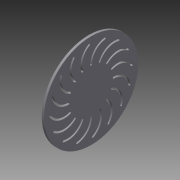
# Autodesk Inventor part: FanCentRotorRear
Saved by Autodesk Inventor 2018.2 (Build 222227000, 227)
## iProperties
Created: 2018-02-04
Part Number: FanCentRotorRear
Material: Generic
Document SubType Name: Sheet Metal
Designer: Rus
Density: 1 g/cm^3
Sheet Metal Rule: Default
Appearance: Default
Author: Rus
Autodesk Inventor part; units mm, degrees
ref_plane "YZ Plane" through (0, 0, 0) normal (1, 0, 0) x (0, 1, 0)
ref_plane "XZ Plane" through (0, 0, 0) normal (0, 1, 0) x (-1, 0, 0)
ref_plane "XY Plane" through (0, 0, 0) normal (0, 0, 1) x (1, 0, 0)
sketch "Sketch1" plane through (0, 0, 0) normal (1, 0, 0) x (0, 1, 0)
  circle A0 centre (0, 0) radius 63.5
  arc A1 (51.7144, -18.8225) -> (30.3724, 0) centre (30.3724, -21.5106) ccw construction
  arc A2 (52.8957, -18.6737) -> (30.3724, 1.1906) centre (30.3724, -21.5106) ccw
  arc A3 (50.5331, -18.9713) -> (30.3724, -1.1906) centre (30.3724, -21.5106) ccw
  arc A4 (50.5331, -18.9713) -> (52.8957, -18.6737) centre (51.7144, -18.8225) ccw
  arc A5 (30.3724, 1.1906) -> (30.3724, -1.1906) centre (30.3724, 0) ccw
  line L0 (51.7144, -18.8225) -> (59.6705, -21.7183) construction
  line L1 (30.3724, 0) -> (63.5, 0) construction
  arc A6 (54.981, 2.4005) -> (28.0605, 11.623) centre (36.2922, -8.2502) ccw construction
  arc A7 (56.0154, 2.99) -> (27.6048, 12.723) centre (36.2922, -8.2502) ccw
  arc A8 (53.9465, 1.811) -> (28.5161, 10.523) centre (36.2922, -8.2502) ccw
  arc A9 (53.9465, 1.811) -> (56.0154, 2.99) centre (54.981, 2.4005) ccw
  arc A10 (27.6048, 12.723) -> (28.5161, 10.523) centre (28.0605, 11.623) ccw
  line L2 (54.981, 2.4005) -> (63.4396, 2.7698) construction
  line L3 (28.0605, 11.623) -> (58.6664, 24.3004) construction
  arc A11 (49.8771, 23.2581) -> (21.4765, 21.4765) centre (36.6869, 6.2662) ccw construction
  arc A12 (50.6072, 24.1986) -> (20.6346, 22.3184) centre (36.6869, 6.2662) ccw
  arc A13 (49.147, 22.3176) -> (22.3184, 20.6346) centre (36.6869, 6.2662) ccw
  arc A14 (49.147, 22.3176) -> (50.6072, 24.1986) centre (49.8771, 23.2581) ccw
  arc A15 (20.6346, 22.3184) -> (22.3184, 20.6346) centre (21.4765, 21.4765) ccw
  line L4 (49.8771, 23.2581) -> (57.5505, 26.8363) construction
  line L5 (21.4765, 21.4765) -> (44.9013, 44.9013) construction
  arc A16 (37.18, 40.5748) -> (11.623, 28.0605) centre (31.4962, 19.8287) ccw construction
  arc A17 (37.4946, 41.7231) -> (10.523, 28.5161) centre (31.4962, 19.8287) ccw
  arc A18 (36.8654, 39.4265) -> (12.723, 27.6048) centre (31.4962, 19.8287) ccw
  arc A19 (36.8654, 39.4265) -> (37.4946, 41.7231) centre (37.18, 40.5748) ccw
  arc A20 (10.523, 28.5161) -> (12.723, 27.6048) centre (11.623, 28.0605) ccw
  line L6 (37.18, 40.5748) -> (42.9, 46.8171) construction
  line L7 (11.623, 28.0605) -> (24.3004, 58.6664) construction
  arc A21 (18.8225, 51.7144) -> (0, 30.3724) centre (21.5106, 30.3724) ccw construction
  arc A22 (18.6737, 52.8957) -> (-1.1906, 30.3724) centre (21.5106, 30.3724) ccw
  arc A23 (18.9713, 50.5331) -> (1.1906, 30.3724) centre (21.5106, 30.3724) ccw
  arc A24 (18.9713, 50.5331) -> (18.6737, 52.8957) centre (18.8225, 51.7144) ccw
  arc A25 (-1.1906, 30.3724) -> (1.1906, 30.3724) centre (0, 30.3724) ccw
  line L8 (18.8225, 51.7144) -> (21.7183, 59.6705) construction
  line L9 (0, 30.3724) -> (0, 63.5) construction
  arc A26 (-2.4005, 54.981) -> (-11.623, 28.0605) centre (8.2502, 36.2922) ccw construction
  arc A27 (-2.99, 56.0154) -> (-12.723, 27.6048) centre (8.2502, 36.2922) ccw
  arc A28 (-1.811, 53.9465) -> (-10.523, 28.5161) centre (8.2502, 36.2922) ccw
  arc A29 (-1.811, 53.9465) -> (-2.99, 56.0154) centre (-2.4005, 54.981) ccw
  arc A30 (-12.723, 27.6048) -> (-10.523, 28.5161) centre (-11.623, 28.0605) ccw
  line L10 (-2.4005, 54.981) -> (-2.7698, 63.4396) construction
  line L11 (-11.623, 28.0605) -> (-24.3004, 58.6664) construction
  arc A31 (-23.2581, 49.8771) -> (-21.4765, 21.4765) centre (-6.2662, 36.6869) ccw construction
  arc A32 (-24.1986, 50.6072) -> (-22.3184, 20.6346) centre (-6.2662, 36.6869) ccw
  arc A33 (-22.3176, 49.147) -> (-20.6346, 22.3184) centre (-6.2662, 36.6869) ccw
  arc A34 (-22.3176, 49.147) -> (-24.1986, 50.6072) centre (-23.2581, 49.8771) ccw
  arc A35 (-22.3184, 20.6346) -> (-20.6346, 22.3184) centre (-21.4765, 21.4765) ccw
  line L12 (-23.2581, 49.8771) -> (-26.8363, 57.5505) construction
  line L13 (-21.4765, 21.4765) -> (-44.9013, 44.9013) construction
  arc A36 (-40.5748, 37.18) -> (-28.0605, 11.623) centre (-19.8287, 31.4962) ccw construction
  arc A37 (-41.7231, 37.4946) -> (-28.5161, 10.523) centre (-19.8287, 31.4962) ccw
  arc A38 (-39.4265, 36.8654) -> (-27.6048, 12.723) centre (-19.8287, 31.4962) ccw
  arc A39 (-39.4265, 36.8654) -> (-41.7231, 37.4946) centre (-40.5748, 37.18) ccw
  arc A40 (-28.5161, 10.523) -> (-27.6048, 12.723) centre (-28.0605, 11.623) ccw
  line L14 (-40.5748, 37.18) -> (-46.8171, 42.9) construction
  line L15 (-28.0605, 11.623) -> (-58.6664, 24.3004) construction
  arc A41 (-51.7144, 18.8225) -> (-30.3724, 0) centre (-30.3724, 21.5106) ccw construction
  arc A42 (-52.8957, 18.6737) -> (-30.3724, -1.1906) centre (-30.3724, 21.5106) ccw
  arc A43 (-50.5331, 18.9713) -> (-30.3724, 1.1906) centre (-30.3724, 21.5106) ccw
  arc A44 (-50.5331, 18.9713) -> (-52.8957, 18.6737) centre (-51.7144, 18.8225) ccw
  arc A45 (-30.3724, -1.1906) -> (-30.3724, 1.1906) centre (-30.3724, 0) ccw
  line L16 (-51.7144, 18.8225) -> (-59.6705, 21.7183) construction
  line L17 (-30.3724, 0) -> (-63.5, 0) construction
  arc A46 (-54.981, -2.4005) -> (-28.0605, -11.623) centre (-36.2922, 8.2502) ccw construction
  arc A47 (-56.0154, -2.99) -> (-27.6048, -12.723) centre (-36.2922, 8.2502) ccw
  arc A48 (-53.9465, -1.811) -> (-28.5161, -10.523) centre (-36.2922, 8.2502) ccw
  arc A49 (-53.9465, -1.811) -> (-56.0154, -2.99) centre (-54.981, -2.4005) ccw
  arc A50 (-27.6048, -12.723) -> (-28.5161, -10.523) centre (-28.0605, -11.623) ccw
  line L18 (-54.981, -2.4005) -> (-63.4396, -2.7698) construction
  line L19 (-28.0605, -11.623) -> (-58.6664, -24.3004) construction
  arc A51 (-49.8771, -23.2581) -> (-21.4765, -21.4765) centre (-36.6869, -6.2662) ccw construction
  arc A52 (-50.6072, -24.1986) -> (-20.6346, -22.3184) centre (-36.6869, -6.2662) ccw
  arc A53 (-49.147, -22.3176) -> (-22.3184, -20.6346) centre (-36.6869, -6.2662) ccw
  arc A54 (-49.147, -22.3176) -> (-50.6072, -24.1986) centre (-49.8771, -23.2581) ccw
  arc A55 (-20.6346, -22.3184) -> (-22.3184, -20.6346) centre (-21.4765, -21.4765) ccw
  line L20 (-49.8771, -23.2581) -> (-57.5505, -26.8363) construction
  line L21 (-21.4765, -21.4765) -> (-44.9013, -44.9013) construction
  arc A56 (-37.18, -40.5748) -> (-11.623, -28.0605) centre (-31.4962, -19.8287) ccw construction
  arc A57 (-37.4946, -41.7231) -> (-10.523, -28.5161) centre (-31.4962, -19.8287) ccw
  arc A58 (-36.8654, -39.4265) -> (-12.723, -27.6048) centre (-31.4962, -19.8287) ccw
  arc A59 (-36.8654, -39.4265) -> (-37.4946, -41.7231) centre (-37.18, -40.5748) ccw
  arc A60 (-10.523, -28.5161) -> (-12.723, -27.6048) centre (-11.623, -28.0605) ccw
  line L22 (-37.18, -40.5748) -> (-42.9, -46.8171) construction
  line L23 (-11.623, -28.0605) -> (-24.3004, -58.6664) construction
  arc A61 (-18.8225, -51.7144) -> (0, -30.3724) centre (-21.5106, -30.3724) ccw construction
  arc A62 (-18.6737, -52.8957) -> (1.1906, -30.3724) centre (-21.5106, -30.3724) ccw
  arc A63 (-18.9713, -50.5331) -> (-1.1906, -30.3724) centre (-21.5106, -30.3724) ccw
  arc A64 (-18.9713, -50.5331) -> (-18.6737, -52.8957) centre (-18.8225, -51.7144) ccw
  arc A65 (1.1906, -30.3724) -> (-1.1906, -30.3724) centre (0, -30.3724) ccw
  line L24 (-18.8225, -51.7144) -> (-21.7183, -59.6705) construction
  line L25 (0, -30.3724) -> (0, -63.5) construction
  arc A66 (2.4005, -54.981) -> (11.623, -28.0605) centre (-8.2502, -36.2922) ccw construction
  arc A67 (2.99, -56.0154) -> (12.723, -27.6048) centre (-8.2502, -36.2922) ccw
  arc A68 (1.811, -53.9465) -> (10.523, -28.5161) centre (-8.2502, -36.2922) ccw
  arc A69 (1.811, -53.9465) -> (2.99, -56.0154) centre (2.4005, -54.981) ccw
  arc A70 (12.723, -27.6048) -> (10.523, -28.5161) centre (11.623, -28.0605) ccw
  line L26 (2.4005, -54.981) -> (2.7698, -63.4396) construction
  line L27 (11.623, -28.0605) -> (24.3004, -58.6664) construction
  arc A71 (23.2581, -49.8771) -> (21.4765, -21.4765) centre (6.2662, -36.6869) ccw construction
  arc A72 (24.1986, -50.6072) -> (22.3184, -20.6346) centre (6.2662, -36.6869) ccw
  arc A73 (22.3176, -49.147) -> (20.6346, -22.3184) centre (6.2662, -36.6869) ccw
  arc A74 (22.3176, -49.147) -> (24.1986, -50.6072) centre (23.2581, -49.8771) ccw
  arc A75 (22.3184, -20.6346) -> (20.6346, -22.3184) centre (21.4765, -21.4765) ccw
  line L28 (23.2581, -49.8771) -> (26.8363, -57.5505) construction
  line L29 (21.4765, -21.4765) -> (44.9013, -44.9013) construction
  arc A76 (40.5748, -37.18) -> (28.0605, -11.623) centre (19.8287, -31.4962) ccw construction
  arc A77 (41.7231, -37.4946) -> (28.5161, -10.523) centre (19.8287, -31.4962) ccw
  arc A78 (39.4265, -36.8654) -> (27.6048, -12.723) centre (19.8287, -31.4962) ccw
  arc A79 (39.4265, -36.8654) -> (41.7231, -37.4946) centre (40.5748, -37.18) ccw
  arc A80 (28.5161, -10.523) -> (27.6048, -12.723) centre (28.0605, -11.623) ccw
  line L30 (40.5748, -37.18) -> (46.8171, -42.9) construction
  line L31 (28.0605, -11.623) -> (58.6664, -24.3004) construction
  dimension "d0" = 127
  dimension "d1" = 20
  dimension "d2" = 8.4667
  dimension "d5" = 2.3813
  dimension "d8" = 360
  dimension "d10" = 20.32
  measures "d0" diameter of A0
  measures "d2" distance of L0.start L0.end
  measures "d5" radial gap between concentric circles of A3 A2
  measures "d10" radius of A3
extrude "Plate1" add sketch "Sketch1" along normal blind 3.048
equation "\"d11\" = Thickness"
equation "\"BendRadius\" = Thickness"
equation "\"BendReliefWidth\" = Thickness"
equation "\"BendReliefDepth\" = 0.5 * Thickness"
equation "\"CornerReliefSize\" = 4 * Thickness"
equation "\"MinimumRemnant\" = 2 * Thickness"
equation "\"TransitionRadius\" = BendRadius"
equation "\"JacobiRadiusSize\" = BendRadius"
equation "\"GapSize\" = Thickness"
equation "\"Thickness\" = 3.048"
body "Solid1"
